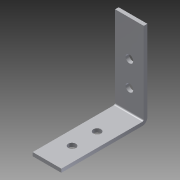
# Autodesk Inventor part: Rebuild Gusset 4
Saved by Autodesk Inventor 2014 SP1 (Build 180222100, 222)
## iProperties
Created: 2013-01-31
Part Number: Rebuild Gusset 4
Material: Aluminum 6061
Document SubType Name: Sheet Metal
Designer: actoennies
Density: 2.71 g/cm^3
Sheet Metal Rule: Default
Mass: 31.1108 g
Surface Area: 86.0215 cm^2
Volume: 11.48 cm^3
Flat Pattern Width: 2.54 cm
Flat Pattern Length: 14.7699 cm
Flat Pattern Area: 37.5156 cm^2
Sheet Metal Width: 1.000 in
Sheet Metal Length: 5.815 in
Sheet Metal Area: 5.815 in^2
Appearance: Aluminum - Flat
Author: actoennies
Autodesk Inventor part; units mm, degrees
note: some values were not read from the file. Left out: dimensions or parameters whose unit could not be read.
ref_plane "YZ Plane" through (0, 0, 0) normal (1, 0, 0) x (0, 1, 0)
ref_plane "XZ Plane" through (0, 0, 0) normal (0, 1, 0) x (-1, 0, 0)
ref_plane "XY Plane" through (0, 0, 0) normal (0, 0, 1) x (1, 0, 0)
sketch "Sketch1" plane through (0, 0, 0) normal (0, 0, 1) x (1, 0, 0)
  line L0 (0, 0) -> (147.699314, 0)
  line L1 (147.699314, -25.4) -> (0, -25.4)
  line L2 (0, 0) -> (73.849657, 0)
  line L3 (73.849657, 0) -> (73.849657, -3.175)
  line L4 (73.849657, -3.175) -> (72.249457, -3.175)
  line L5 (72.249457, -3.175) -> (72.249457, -9.525)
  line L6 (72.249457, -9.525) -> (75.424457, -9.525)
  line L7 (75.424457, -9.525) -> (75.424457, -3.175)
  line L8 (75.424457, -3.175) -> (73.849657, -3.175)
  line L9 (73.849657, -25.4) -> (73.849657, -22.225)
  line L10 (73.849657, -22.225) -> (72.249457, -22.225)
  line L11 (72.249457, -22.225) -> (72.249457, -15.875)
  line L12 (72.249457, -15.875) -> (75.424457, -15.875)
  line L13 (75.424457, -15.875) -> (75.424457, -22.225)
  line L14 (75.424457, -22.225) -> (73.849657, -22.225)
  dimension "d8" = 6.7564
sketch "Sketch3" plane through (0, 3.175, 76.2) normal (0, 1, 0) x (1, 0, 0)
  line L0 (0, 0) -> (25.4, 0) projected
  circle A0 centre (12.7, 44.45) radius 3.3782
  circle A1 centre (12.7, 22.225) radius 3.3782
  line L1 (0, 76.2) -> (0, 73.025) projected
  dimension "d21" = 6.7564
  dimension "d22" = 6.7564
  dimension "d23" = 12.7
  dimension "d24" = 22.225
  dimension "d25" = 22.225
  constraints: 2 centre point
  measures "d21" diameter of A0
  measures "d22" diameter of A1
  measures "d23" distance from line of L1 A0.centre
  measures "d24" distance from line of L0 A1.centre
  measures "d25" distance of A1.centre A0.centre
sketch "Sketch1 outline for Plate1" plane through (0, 0, 0) normal (0, 0, 1) x (1, 0, 0)
  line L0 (0, 0) -> (0, 76.2)
  line L1 (25.4, 0) -> (0, 0)
  line L2 (0, 76.2) -> (25.4, 76.2)
  line L3 (25.4, 76.2) -> (25.4, 0)
  circle A0 centre (12.7, 22.225) radius 3.3782
  circle A1 centre (12.7, 44.45) radius 3.3782
extrude "Plate1" add sketch "Sketch1 outline for Plate1" along normal blind 3.175
sketch "Sketch2" plane through (25.4, 3.175, 0) normal (0, -1, 0) x (1, 0, 0)
  line L0 (-25.4, 0) -> (0, 0)
  line L1 (0, 0) -> (0, 76.2)
  line L2 (0, 76.2) -> (-25.4, 76.2)
  line L3 (-25.4, 76.2) -> (-25.4, 0)
  constraints: 6 end point, 1 horizontal, 1 perpendicular, 1 vertical
edge flange "Flange1" height 76.2 angle 90 thickness 3.175 bend radius 1.27 thickness toward (0, -1, 0) relief tear relief width 3.175 relief depth 1.5875 edges at (12.7, 0, 3.175) wall of the first edge with corners at (0, 3.175, 0) (25.4, 3.175, 0) (25.4, 3.175, 76.2) (0, 3.175, 76.2)
bend "Bend1"
corner "Corner1"
extrude "Cut1" cut sketch "Sketch3" against normal blind 3.175
equation "\"d11\" = BendReliefWidth"
equation "\"d12\" = BendReliefDepth"
equation "\"d13\" = MinimumRemnant"
equation "\"d14\" = BendRadius"
equation "\"d18\" = CornerReliefSize"
equation "\"d19\" = GapSize"
equation "\"d20\" = JacobiRadiusSize"
equation "\"BendRadius\" = Thickness"
equation "\"BendReliefWidth\" = Thickness"
equation "\"BendReliefDepth\" = 0.5 * Thickness"
equation "\"CornerReliefSize\" = 4 * Thickness"
equation "\"MinimumRemnant\" = 2 * Thickness"
equation "\"TransitionRadius\" = BendRadius"
equation "\"JacobiRadiusSize\" = BendRadius"
equation "\"GapSize\" = Thickness"
equation "\"d10\" = BendRadius"
equation "\"d6\" = Thickness"
equation "\"Thickness\" = 3.175"
body "Solid1"
